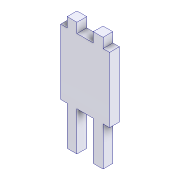
# Autodesk Inventor part: motor_stick
Saved by Autodesk Inventor 2020 (Build 240168000, 168)
## iProperties
Created: 2021-05-10
Part Number: motor_stick
Material: Generic
Document SubType Name: Modeling
Designer: Hsu Daniel
Density: 1 g/cm^3
Appearance: Cool White
Author: Hsu Daniel
Autodesk Inventor part; units mm, degrees
ref_plane "YZ Plane" through (0, 0, 0) normal (1, 0, 0) x (0, 1, 0)
ref_plane "XZ Plane" through (0, 0, 0) normal (0, 1, 0) x (-1, 0, 0)
ref_plane "XY Plane" through (0, 0, 0) normal (0, 0, 1) x (1, 0, 0)
sketch "Sketch1" plane through (0, 0, 0) normal (0, 0, 1) x (1, 0, 0)
  line L0 (0, 0) -> (2, 0)
  line L1 (2, 0) -> (2, -12)
  line L2 (2, -12) -> (5, -12)
  line L3 (5, -12) -> (5, 0)
  line L4 (5, 0) -> (10, 0)
  line L5 (10, 0) -> (10, -12)
  line L6 (10, -12) -> (13, -12)
  line L7 (13, -12) -> (13, 0)
  line L8 (13, 0) -> (15, 0)
  line L9 (15, 0) -> (15, 20)
  line L10 (15, 20) -> (13, 20)
  line L11 (13, 20) -> (13, 23)
  line L12 (13, 23) -> (10, 23)
  line L13 (10, 23) -> (10, 20)
  line L14 (5, 20) -> (5, 23)
  line L15 (5, 20) -> (10, 20)
  line L16 (5, 23) -> (2, 23)
  line L17 (2, 23) -> (2, 20)
  line L18 (2, 20) -> (0, 20)
  line L19 (0, 20) -> (0, 0)
  line L20 (3.5, -12) -> (3.5, 6.8939) construction
  line L21 (7.5, 0) -> (7.5, 4.8399) construction
  dimension "d0" = 2
  dimension "d1" = 12
  dimension "d2" = 3
  dimension "d3" = 3
  dimension "d4" = 2
  dimension "d5" = 3
  dimension "d8" = 20
  dimension "d11" = 4
  constraints: 44 end point, 20 point on line, 9 perpendicular, 2 midpoint, 2 vertical, 1 horizontal
  measures "d0" distance of L0.start L0.end
  measures "d1" distance of L0.end L1.end
  measures "d2" distance of L1.end L2.end
  measures "d3" distance of L5.end L6.end
  measures "d4" distance of L7.end L8.end
  measures "d5" distance of L10.end L11.end
  measures "d8" distance of L8.end L9.end
  measures "d11" distance between parallel lines of L20 L21
extrude "Extrusion1" add sketch "Sketch1" along normal blind 3
equation "\"d4\" = d0"
body "Solid1"
